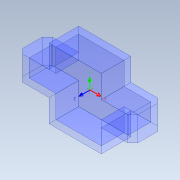
# Autodesk Inventor part: body
Saved by Autodesk Inventor 2020 (Build 240168000, 168)
## iProperties
Created: 2021-01-12
Part Number: body
Material: Generic
Document SubType Name: Modeling
Designer: DELL
Density: 1 g/cm^3
Appearance: Clear - Blue
Author: DELL
Autodesk Inventor part; units mm, degrees
ref_plane "YZ Plane" through (0, 0, 0) normal (1, 0, 0) x (0, 1, 0)
ref_plane "XZ Plane" through (0, 0, 0) normal (0, 1, 0) x (-1, 0, 0)
ref_plane "XY Plane" through (0, 0, 0) normal (0, 0, 1) x (1, 0, 0)
sketch "Sketch1" plane through (0, 0, 0) normal (0, 0, 1) x (1, 0, 0)
  line L0 (75, -100) -> (-75, -100)
  line L1 (-75, 100) -> (75, 100)
  line L2 (75, -100) -> (-75, 100) construction
  line L3 (-75, -100) -> (75, 100) construction
  line L4 (-165, -35) -> (-165, 35)
  line L5 (165, 35) -> (165, -35)
  line L6 (165, -35) -> (-165, 35) construction
  line L7 (-165, -35) -> (165, 35) construction
  line L8 (-75, -100) -> (-75, -35)
  line L9 (-75, 35) -> (-75, 100)
  line L10 (-165, 35) -> (-75, 35)
  line L11 (75, 35) -> (165, 35)
  line L12 (75, 100) -> (75, 35)
  line L13 (75, -35) -> (75, -100)
  line L14 (165, -35) -> (75, -35)
  line L15 (-75, -35) -> (-165, -35)
  line L16 (-65, 90) -> (65, 90)
  line L17 (65, 90) -> (65, 25)
  line L18 (65, 25) -> (155, 25)
  line L19 (155, 25) -> (155, -25)
  line L20 (155, -25) -> (65, -25)
  line L21 (65, -25) -> (65, -90)
  line L22 (65, -90) -> (-65, -90)
  line L23 (-65, -90) -> (-65, -25)
  line L24 (-65, -25) -> (-155, -25)
  line L25 (-155, -25) -> (-155, 25)
  line L26 (-155, 25) -> (-65, 25)
  line L27 (-65, 25) -> (-65, 90)
  line L28 (-142, 25) -> (-142, -25)
  line L29 (142, 25) -> (142, -25)
  point P0 (0, 0)
  point P1 (0, 0)
  point P2 (0, 0)
  point P3 (0, 0)
  point P4 (0, 0)
  dimension "d0" = 70
  dimension "d1" = 330
  dimension "d2" = 150
  dimension "d3" = 200
  dimension "d10" = 10
  dimension "d11" = 23
  dimension "d12" = 23
  constraints: 60 end point, 20 parallel, 10 perpendicular, 8 collinear, 6 midpoint, 4 point on line, 3 horizontal, 2 coincident, 11 other
  measures "d0" distance of L5.start L5.end
  measures "d1" distance of L5.end L4.start
  measures "d2" distance of L0.start L0.end
  measures "d3" distance of L1.end L0.start
  measures "d10" distance between parallel lines of L9 L27
  measures "d11" distance between parallel lines of L4 L28
  measures "d12" distance between parallel lines of L5 L29
extrude "Extrusion1" add sketch "Sketch1" along normal mid plane 85 contours L0 L8 L15 L4 L10 L9 L1 L12 L11 L5 L14 L13 | L16 L17 L18 L29 L20 L21 L22 L23 L24 L28 L26 L27 | L28 L24 L25 L26 | L18 L19 L20 L29
sketch "Sketch2" plane through (0, 0, 0) normal (0, 1, 0) x (-1, 0, 0)
  line L0 (-150, 42.5) -> (-165, 27.5)
  line L1 (-165, -42.5) -> (-165, 42.5) projected
  line L2 (-165, -27.5) -> (-150, -42.5)
  line L3 (-165, -42.5) -> (-75, -42.5) projected
  line L4 (75, 42.5) -> (165, 42.5) projected
  line L5 (150, 42.5) -> (165, 27.5)
  line L6 (165, -42.5) -> (165, 42.5) projected
  line L7 (-165, -42.5) -> (165, -42.5) projected
  line L8 (150, -42.5) -> (165, -27.5)
  line L9 (-165, 42.5) -> (165, 42.5) projected
  line L10 (165, 0) -> (-165, 0) construction
  line L11 (-165, 42.5) -> (-165, -42.5) construction
  line L12 (-75, 42.5) -> (75, 42.5) construction
  line L13 (0, 42.5) -> (0, -42.5) construction
  line L14 (75, -42.5) -> (-75, -42.5) construction
  point P0 (0, 0)
  dimension "d6" = 15
  dimension "d7" = 45
  constraints: 12 end point, 8 point on line, 4 midpoint, 3 perpendicular, 2 other
  measures "d6" horizontal distance of L0.start L0.end
  measures "d7" angle of L1 L0
extrude "Extrusion2" cut sketch "Sketch2" along normal through all both and the other way through all contours L0 L1 L9 | L2 L3 L1 | L4 L6 L5 | L6 L7 L8
extrude "Extrusion3" cut sketch "Sketch1" along normal mid plane 65 contours L16 L17 L18 L29 L20 L21 L22 L23 L24 L28 L26 L27
equation "\"d10\" = wall_thickness"
equation "\"d13\" = body_thickness - 2 * wall_thickness"
equation "\"wall_thickness\" = 10"
equation "\"body_thickness\" = 85"
body "Solid1"
